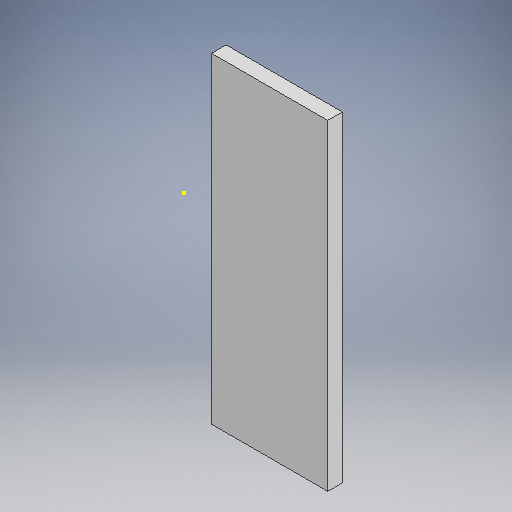
# Autodesk Inventor part: Lifting Sections floor
Saved by Autodesk Inventor 2025.3 (Build 293356000, 356)
## iProperties
Created: 2026-04-06
Part Number: Lifting Sections floor
Material: Generic
Document SubType Name: Modeling
Designer: user
Density: 1 g/cm^3
Appearance: Default
Author: user
Autodesk Inventor part; units mm, degrees
ref_plane "YZ Plane" through (0, 0, 0) normal (1, 0, 0) x (0, 1, 0)
ref_plane "XZ Plane" through (0, 0, 0) normal (0, 1, 0) x (-1, 0, 0)
ref_plane "XY Plane" through (0, 0, 0) normal (0, 0, 1) x (1, 0, 0)
sketch "Sketch1" plane through (0, 0, 0) normal (0, 0, 1) x (1, 0, 0)
  point P0 (0, 0)
sketch "Sketch2" plane through (0, 0, 0) normal (0, 0, 1) x (1, 0, 0)
  line L0 (14.3533, -58.9008) -> (54.1533, -58.9008)
  line L1 (54.1533, -58.9008) -> (54.1533, 51.0992)
  line L2 (54.1533, 51.0992) -> (14.3533, 51.0992)
  line L3 (14.3533, 51.0992) -> (14.3533, -58.9008)
  line L4 (54.1533, -3.9008) -> (14.3533, -3.9008) construction
  line L5 (54.1533, 51.0992) -> (54.1533, 36.0992)
  line L6 (54.1533, 26.0992) -> (54.1533, 36.0992)
  line L7 (34.2533, 51.0992) -> (34.2533, -58.9008) construction
  dimension "d1" = 39.8
  dimension "d2" = 110
  constraints: 16 end point, 4 midpoint, 2 parallel, 1 collinear, 1 horizontal, 1 perpendicular
  measures "d1" distance of L2.start L2.end
  measures "d2" distance of L1.start L2.start
extrude "Extrusion1" add sketch "Sketch2" along normal blind 5
body "Solid1"
